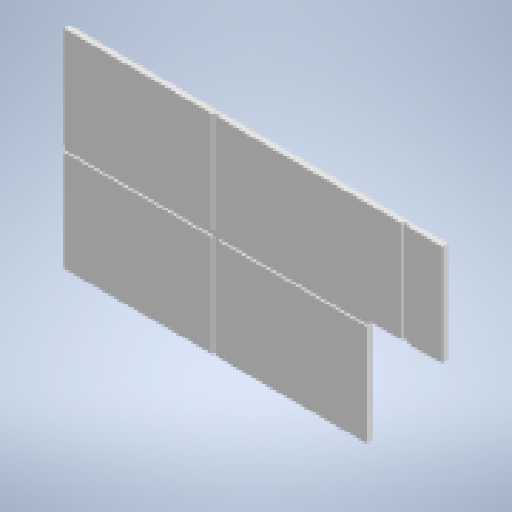
# Autodesk Inventor part: Wire Position
Saved by Autodesk Inventor 2025.2 (Build 292293000, 293)
## iProperties
Created: 2025-04-29
Part Number: Wire Position
Material: Generic
Document SubType Name: Modeling
Designer: powel
Density: 1 g/cm^3
Appearance: Default
Author: powel
Autodesk Inventor part; units mm, degrees
ref_plane "YZ Plane" through (0, 0, 0) normal (1, 0, 0) x (0, 1, 0)
ref_plane "XZ Plane" through (0, 0, 0) normal (0, 1, 0) x (-1, 0, 0)
ref_plane "XY Plane" through (0, 0, 0) normal (0, 0, 1) x (1, 0, 0)
sketch "Sketch1" plane through (0, 0, 0) normal (0, 0, 1) x (1, 0, 0)
  line L0 (0, 0) -> (32, 0)
  line L1 (32, 0) -> (32, 22)
  line L2 (32, 22) -> (0, 22)
  line L3 (0, 22) -> (0, 0)
  line L4 (0, 11) -> (0, 10.7)
  line L5 (0, 10.7) -> (0, 11.3)
  line L6 (32, 16.3) -> (32, 15.7)
  line L7 (0, 15.7) -> (0, 11.3)
  line L8 (16.3, 22) -> (15.7, 22)
  line L9 (15.7, 22) -> (16.3, 22)
  line L10 (16.3, 0) -> (15.7, 0)
  line L11 (32, 11) -> (32, 11.3)
  line L12 (0, 11.3) -> (0, 10.7)
  line L13 (32, 10.7) -> (32, 11.3)
  line L14 (16.3, 22) -> (15.7, 22)
  line L15 (15.7, 0) -> (16.3, 0)
  line L16 (0, 10.7) -> (15.7, 10.7)
  line L17 (16.3, 10.7) -> (32, 10.7)
  line L18 (16.3, 0) -> (16.3, 10.7)
  line L19 (16.3, 11.3) -> (16.3, 22)
  line L20 (32, 11.3) -> (16.3, 11.3)
  line L21 (15.7, 11.3) -> (0, 11.3)
  line L22 (15.7, 22) -> (15.7, 11.3)
  line L23 (15.7, 10.7) -> (15.7, 0)
  line L24 (32, 11.3) -> (40, 11.3)
  line L25 (40, 11.3) -> (40, 22)
  line L26 (40, 22) -> (32, 22)
  line L27 (32, 22) -> (32, 11.3)
  line L28 (36, 22) -> (36.3, 22)
  line L29 (36.3, 22) -> (35.7, 22)
  line L30 (35.7, 22) -> (35.7, 11.3)
  line L31 (35.7, 11.3) -> (36.3, 11.3)
  line L32 (36.3, 11.3) -> (36.3, 22)
  point P0 (36.3, 16.3)
  dimension "d1" = 22
  dimension "d6" = 0.6
  dimension "d14" = 0.3
  dimension "d15" = 0.6
  dimension "d16" = 0.6
  dimension "d17" = 8
  dimension "d18" = 0.3
  dimension "d19" = 0.6
  constraints: 66 end point, 18 parallel, 8 point on line, 7 horizontal, 7 perpendicular, 3 midpoint
  measures "d1" distance of L2.end L0.start
  measures "d6" distance of L8.end L8.start
  measures "d14" distance of L11.start L11.end
  measures "d15" distance of L5.start L12.start
  measures "d16" distance of L15.end L10.end
  measures "d17" distance of L26.end L25.end
  measures "d18" distance of L28.start L28.end
  measures "d19" distance of L31.end L30.end
extrude "Extrusion1" add sketch "Sketch1" against normal blind 0.4
extrude "Extrusion2" add sketch "Sketch1" along normal blind 0.2 contours L3 L16 L23 L0 | L18 L17 L1 L0 | L3 L2 L22 L21 | L20 L19 L2 L1 | L1 L26 L30 L24 | L32 L26 L25 L24
body "Solid1"
